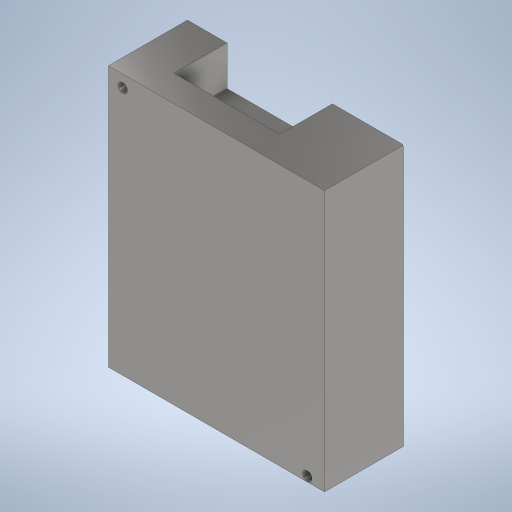
# Autodesk Inventor part: PSU
Saved by Autodesk Inventor 2024 (Build 280153000, 153)
## iProperties
Created: 2026-05-31
Part Number: PSU
Material: Stahl, weich
Document SubType Name: Modeling
Designer: maxim
Density: 7.85 g/cm^3
Appearance: Halbpoliert
Author: maxim
Autodesk Inventor part; units mm, degrees
ref_plane "YZ Plane" through (0, 0, 0) normal (1, 0, 0) x (0, 1, 0)
ref_plane "XZ Plane" through (0, 0, 0) normal (0, 1, 0) x (-1, 0, 0)
ref_plane "XY Plane" through (0, 0, 0) normal (0, 0, 1) x (1, 0, 0)
sketch "Skizze1" plane through (0, 0, 0) normal (0, 1, 0) x (-1, 0, 0)
  line L0 (0, 0) -> (82, 0)
  line L1 (82, 0) -> (82, -99)
  line L2 (82, -99) -> (0, -99)
  line L3 (0, -99) -> (0, 0)
  dimension "d0" = 82
  dimension "d1" = 99
  constraints: 8 end point, 2 parallel, 1 horizontal, 1 perpendicular
  measures "d0" distance of L1.end L2.end
  measures "d1" distance of L0.end L1.end
extrude "Extrusion1" add sketch "Skizze1" along normal blind 30
sketch "Skizze2" plane through (0, 30, 0) normal (0, 1, 0) x (1, 0, 0)
  point P0 (0, 0)
sketch "Skizze3" plane through (0, 30, 0) normal (0, 1, 0) x (1, 0, 0)
  line L0 (-82, 0) -> (0, 0) projected
  line L1 (0, 0) -> (0, 99) projected
  point P0 (-76.5, 4.5)
  point P1 (-6.5, 97)
  dimension "d4" = 4.5
  dimension "d5" = 92.5
  dimension "d7" = 6.5
  dimension "d8" = 70
  measures "d4" distance from line of L0 point (-76.5, 4.5)
  measures "d5" vertical distance of point (-6.5, 97) point (-76.5, 4.5)
  measures "d7" distance from line of L1 point (-6.5, 97)
  measures "d8" horizontal distance of point (-76.5, 4.5) point (-6.5, 97)
hole "Bohrung1" at (-76.5, 30, -4.5) at (-6.5, 30, -97) direction (0, -1, 0) diameter 3.5 end through all
sketch "Skizze4" plane through (0, 30, 0) normal (0, 1, 0) x (1, 0, 0)
  line L0 (-82, 0) -> (0, 0) projected
  line L1 (-67, 0) -> (-27, 0)
  line L2 (-27, 0) -> (-27, 15)
  line L3 (-27, 15) -> (-67, 15)
  line L4 (-67, 15) -> (-67, 0)
  line L5 (-82, 99) -> (-82, 0) projected
  dimension "d16" = 15
  dimension "d17" = 15
  dimension "d18" = 40
  constraints: 8 end point, 2 parallel, 2 point on line, 1 perpendicular
  measures "d16" distance between parallel lines of L5 L4
  measures "d17" distance of L3.end L1.start
  measures "d18" distance of L2.end L3.end
extrude "Extrusion2" cut sketch "Skizze4" against normal blind 20
